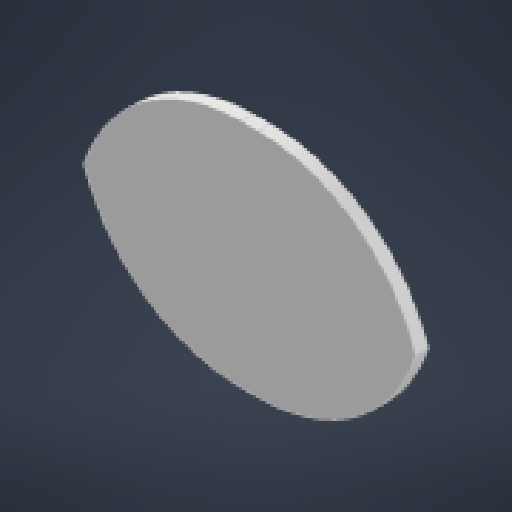
# Autodesk Inventor part: Part2
Saved by Autodesk Inventor 2027 (Build 310192060, 192F)
## iProperties
Created: 2026-08-17
Part Number: Part2
Material: Generic
Document SubType Name: Modeling
Designer: trtrn
Density: 1 g/cm^3
Appearance: Default
Author: trtrn
Autodesk Inventor part; units mm, degrees
ref_plane "YZ Plane" through (0, 0, 0) normal (1, 0, 0) x (0, 1, 0)
ref_plane "XZ Plane" through (0, 0, 0) normal (0, 1, 0) x (-1, 0, 0)
ref_plane "XY Plane" through (0, 0, 0) normal (0, 0, 1) x (1, 0, 0)
sketch "Sketch1" plane through (0, 0, 0) normal (0, 0, 1) x (1, 0, 0)
  line L0 (-40, 40) -> (40, 40)
  line L1 (40, 40) -> (40, -40)
  line L2 (40, -40) -> (-40, -40)
  line L3 (-40, -40) -> (-40, 40)
  line L4 (-40, 40) -> (40, -40) construction
  line L5 (40, 40) -> (-40, -40) construction
  point P0 (0, 0)
  dimension "d0" = 80
  dimension "d1" = 80
  constraints: 12 end point, 2 midpoint, 2 parallel, 1 horizontal, 1 perpendicular
  measures "d0" distance of L1.end L2.end
  measures "d1" distance of L0.end L1.end
extrude "Extrusion1" add sketch "Sketch1" along normal blind 3
sketch "Sketch2" plane through (0, 0, 3) normal (0, 0, 1) x (1, 0, 0)
  arc A0 (-2, 26.8827) -> (-40, -0.967) centre (-2, -12.967) ccw projected
  arc A1 (40, -0.967) -> (2, 26.8827) centre (2, -12.967) ccw projected
  line L0 (2, 26.8827) -> (-2, 26.8827) projected
  line L1 (-40, -0.967) -> (40, -0.967) construction
  line L2 (40, -40) -> (40, 40) construction
  arc A2 (-2, 26.8827) -> (-40, -0.967) centre (-2, -12.967) ccw construction
  arc A3 (40, -0.967) -> (2, 26.8827) centre (2, -12.967) ccw construction
  arc A4 (-2, 26.8827) -> (-40, -0.967) centre (-2, -12.967) ccw
  arc A5 (40, -0.967) -> (2, 26.8827) centre (2, -12.967) ccw
  line L3 (-2, 26.8827) -> (2, 26.8827)
  arc A6 (-2, 26.8827) -> (-40, -0.967) centre (-2, -12.967) ccw
  arc A7 (40, -0.967) -> (2, 26.8827) centre (2, -12.967) ccw
  line L4 (2, 26.8827) -> (-2, 26.8827)
  arc A8 (-40, -0.967) -> (-2, -28.8167) centre (-2, 11.033) ccw
  arc A9 (2, -28.8167) -> (40, -0.967) centre (2, 11.033) ccw
  line L5 (2, -28.8167) -> (-2, -28.8167)
  line L6 (-40, 40) -> (-40, -40) projected
  line L7 (-40, -0.967) -> (-40, 40)
  line L8 (40, 40) -> (-40, 40) projected
  line L9 (-40, 40) -> (40, 40)
  line L10 (40, 40) -> (40, -0.967)
  line L11 (40, -0.967) -> (40, -40)
  line L12 (-40, -40) -> (40, -40) projected
  line L13 (-40, -40) -> (40, -40)
  line L14 (40, -40) -> (-40, -40)
  point P0 (0, 0)
  constraints: 20 end point, 16 point on circle, 8 centre point, 5 collinear, 5 concentric, 4 symmetric about line, 2 perpendicular, 1 horizontal, 2 other
extrude "Extrusion2" cut sketch "Sketch2" against normal blind 3 contours A0 L6 L8 L10 A1 L0 | A8 L5 A9 L11 L12 L6
sketch "Sketch3" plane through (0, 0, 3) normal (0, 0, 1) x (1, 0, 0)
  circle A0 centre (0, -0.967) radius 16 projected
  point P0 (0, 0)
extrude "Extrusion3" cut sketch "Sketch3" against normal blind 3
body "Solid1"
